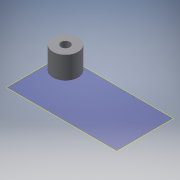
# Autodesk Inventor part: roller
Saved by Autodesk Inventor 2018 (Build 220112000, 112)
## iProperties
Created: 2017-11-13
Part Number: roller
Material: Generic
Document SubType Name: Modeling
Designer: leo2a
Density: 1 g/cm^3
Appearance: Default
Author: leo2a
Autodesk Inventor part; units mm, degrees
ref_plane "YZ Plane" through (0, 0, 0) normal (1, 0, 0) x (0, 1, 0)
ref_plane "XZ Plane" through (0, 0, 0) normal (0, 1, 0) x (-1, 0, 0)
ref_plane "XY Plane" through (0, 0, 0) normal (0, 0, 1) x (1, 0, 0)
ref_plane "Work Plane1" through (-8.2554, -4.8381, 0.5113) normal (0, 0, -1) x (-1, 0, 0)
sketch "Sketch1" plane through (-8.2554, -4.8381, 0.5113) normal (0, 0, -1) x (-1, 0, 0)
  line L0 (0, 0) -> (1.75, 0)
  line L1 (1.75, 0) -> (1.75, 3)
  circle A0 centre (1.75, 3) radius 0.8
  circle A1 centre (1.75, 3) radius 2.25
  point P0 (-8.2554, 4.8381)
  dimension "d0" = 1.75
  dimension "d1" = 3
  dimension "d2" = 1.6
  dimension "d3" = 4.5
  constraints: 4 end point, 2 centre point, 2 coincident, 1 horizontal, 1 perpendicular
  measures "d0" distance of L0.start L0.end
  measures "d1" distance of L0.end L1.end
  measures "d2" diameter of A0
  measures "d3" diameter of A1
extrude "Extrusion1" add sketch "Sketch1" against normal blind 4
body "Solid1"
